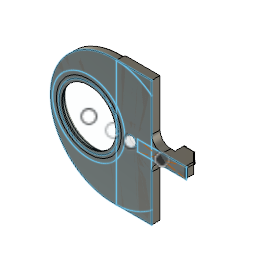
52mm filter holder (Autodesk Fusion 360 design; units mm, degrees)
Autodesk Fusion 360 part; units mm, degrees
other "Base Mesh Feature1"
sketch "Sketch1" plane through (0, 0, 0) normal (1, 0, 0) x (0, 1, 0)
sketch "Sketch2" plane through (0, 0, 0) normal (0, 1, 0) x (1, 0, 0)
  line L0 (61.452474, -115.997991) -> (93.991658, -115.997991)
  line L1 (93.991658, -115.997991) -> (93.991658, -0.000968)
  line L2 (93.991658, -0.000968) -> (61.452474, -0.000968)
  line L3 (61.452474, -0.000968) -> (61.452474, -115.997991)
  arc A0 (93.991658, -12.144928) -> (93.991658, -103.854032) centre (58.342548, -57.99948) ccw
  circle A1 centre (75.007736, -57.988843) radius 4.489901
  circle A2 centre (35.846582, -57.916383) radius 33.452473
  circle A3 centre (35.846582, -57.916383) radius 27.5
  dimension "d1" = 55
  constraint perpendicular L0 L1
  constraint parallel L0 L2
  constraint parallel L1 L3
  constraint horizontal L0
  constraint concentric A2 A3
  measures "d1" diameter of A3
sketch "Sketch3" plane through (0, 0, 0) normal (0, 1, 0) x (1, 0, 0)
  line L0 (81.123679, -52.444918) -> (126.123679, -52.444918)
  line L1 (126.123679, -52.444918) -> (126.123679, -62.444918)
  line L2 (126.123679, -62.444918) -> (81.123679, -62.444918)
  line L3 (81.123679, -62.444918) -> (81.123679, -52.444918)
  line L4 (81.123679, -52.444918) -> (126.123679, -62.444918) construction
  line L5 (126.123679, -52.444918) -> (81.123679, -62.444918) construction
  point P0 (103.623679, -57.444918)
  dimension "d2" = 45
  dimension "d3" = 10
  constraint horizontal L0
  constraint perpendicular L0 L1
  constraint parallel L0 L2
  constraint parallel L1 L3
extrude "Extrude1" add sketch "Sketch3" sketch "Sketch2" along normal blind 7.75 contours L0 L1 L2 L3 picked at (96.123679, -59.111585) of sketch 2 contours L0 L1 A0 | L3 A0 A2 | L1 L3 A0 A2 | L3 A2 A3 | L3 A2 A3 | L1 L2 A0 picked at (92.052301, -109.229105) picked at (54.685817, -106.726274) picked at (89.160318, -57.995934) picked at (58.004249, -35.668658) picked at (65.283815, -68.878298) picked at (92.052301, -6.769855) makes body 1
sketch "Sketch4" plane through (0, 0, 0) normal (0, 1, 0) x (1, 0, 0)
  circle A0 centre (35.831406, -57.884516) radius 25
  circle A1 centre (35.831406, -57.884516) radius 30
  dimension "d6" = 50
  dimension "d7" = 5
  measures "d6" diameter of A0
extrude "Extrude2" add sketch "Sketch4" along normal blind 1 separate body contours A1 picked at (64.053048, -59.374939) makes body 2
chamfer "Chamfer1" distance 1 distance2 4.5 1 edges at (70.821679, 7.75, 56.365225) measured on face at (70.483213, 7.75, 102.872372) on bodies 1
sketch "Sketch5" plane through (0, 7.75, 0) normal (0, 1, 0) x (-1, 0, 0)
  circle A0 centre (-35.846582, 57.916383) radius 27.5
  line L0 (-93.991658, 62.444918) -> (-126.123679, 62.444918)
  line L1 (-126.123679, 62.444918) -> (-126.123679, 52.444918)
  line L2 (-126.123679, 52.444918) -> (-93.991658, 52.444918)
  line L3 (-93.991658, 52.444918) -> (-93.991658, 0.000968)
  line L4 (-93.991658, 0.000968) -> (-61.452474, 0.000968)
  arc A1 (-61.452474, 0.000968) -> (-61.452474, 115.997991) centre (-58.342548, 57.99948) ccw
  line L5 (-61.452474, 115.997991) -> (-93.991658, 115.997991)
  line L6 (-93.991658, 115.997991) -> (-93.991658, 62.444918)
  circle A2 centre (-75.007736, 57.988843) radius 5.489901
  line L7 (-126.123679, 62.444918) -> (-122.123679, 62.444918)
  line L8 (-122.123679, 62.444918) -> (-122.123679, 51.688197)
  line L9 (-122.123679, 51.688197) -> (-126.123679, 51.688197)
  line L10 (-126.123679, 51.688197) -> (-126.123679, 62.444918)
  dimension "d12" = 4
  constraint horizontal L7
  constraint vertical L8
  constraint horizontal L9
  constraint vertical L10
fillet "Fillet1" radius 3 1 edges at (10.20758, 7.75, 47.971959) on bodies 1
fillet "Fillet2" radius 1 1 edges at (69.889352, 7.75, 59.974076) on bodies 1
fillet "Fillet3" radius 2 1 edges at (0.260718, 7.75, 57.99948) on bodies 1
sketch "Sketch7" plane through (0, 7.75, 0) normal (0, 1, 0) x (-1, 0, 0)
  arc A0 (-63.452474, 115.997991) -> (-61.345386, 114.00086) centre (-61.452474, 115.997991) ccw
  line L0 (-63.452474, 115.997991) -> (-93.991658, 115.997991)
  line L1 (-93.991658, 115.997991) -> (-93.991658, 62.444918)
  line L2 (-93.991658, 62.444918) -> (-126.123679, 62.444918)
  line L3 (-126.123679, 62.444918) -> (-126.123679, 52.444918)
  line L4 (-126.123679, 52.444918) -> (-93.991658, 52.444918)
  line L5 (-93.991658, 52.444918) -> (-93.991658, 0.000968)
  line L6 (-93.991658, 0.000968) -> (-63.452474, 0.000968)
  arc A1 (-61.345386, 1.998099) -> (-63.452474, 0.000968) centre (-61.452474, 0.000968) ccw
  arc A2 (-61.345386, 1.998099) -> (-61.345386, 114.00086) centre (-58.342548, 57.99948) ccw
  circle A3 centre (-35.846582, 57.916383) radius 30.5
  circle A4 centre (-75.007736, 57.988843) radius 6.292072
  line L7 (-117.844827, 62.444918) -> (-107.844827, 62.444918)
  line L8 (-107.844827, 62.444918) -> (-107.844827, 52.444918)
  line L9 (-107.844827, 52.444918) -> (-117.844827, 52.444918)
  line L10 (-117.844827, 52.444918) -> (-117.844827, 62.444918)
  dimension "d27" = 10
  dimension "d28" = 10
  constraint horizontal L7
  constraint vertical L8
  constraint horizontal L9
  constraint vertical L10
extrude "Extrude4" add sketch "Sketch7" along normal blind 10 contours L2 L4 L7 L8 L9 L10 picked at (-114.511494, 55.778252) bodies 1
chamfer "Chamfer2" distance 7 angle 45 1 edges at (117.844827, 7.75, 57.444918) on bodies 1
fillet "Fillet7" radius 2 1 faces at (114.511494, 17.75, 55.778252) on bodies 1
fillet "Fillet8" radius 1 1 faces at (126.123679, 2.583333, 55.778252) on bodies 1
fillet "Fillet9" radius 10 1 edges at (93.991658, 3.875, 52.444918) on bodies 1
fillet "Fillet10" radius 10 1 edges at (93.991658, 3.875, 62.444918) on bodies 1
